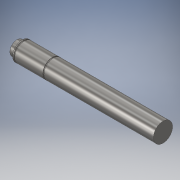
# Autodesk Inventor part: Main Axle
Saved by Autodesk Inventor 2019.4 (Build 234330000, 330)
## iProperties
Created: 2019-11-02
Part Number: Main Axle
Material: Stainless Steel
Document SubType Name: Modeling
Designer: admin
Density: 8 g/cm^3
Appearance: Semi-Polished
Author: admin
Autodesk Inventor part; units mm, degrees
ref_plane "YZ Plane" through (0, 0, 0) normal (1, 0, 0) x (0, 1, 0)
ref_plane "XZ Plane" through (0, 0, 0) normal (0, 1, 0) x (-1, 0, 0)
ref_plane "XY Plane" through (0, 0, 0) normal (0, 0, 1) x (1, 0, 0)
sketch "Sketch1" plane through (0, 0, 0) normal (0, 1, 0) x (-1, 0, 0)
  line L0 (0, 0) -> (0, -7.3)
  line L1 (0, -7.3) -> (-5.3, -7.3)
  line L2 (-5.3, -7.3) -> (-5.3, -9.8)
  line L3 (-150, -9.8) -> (-150, 0)
  line L4 (-150, 0) -> (0, 0)
  line L5 (-5.3, -9.8) -> (-6.4, -9.8)
  line L6 (-6.4, -9.8) -> (-6.4, -9.3)
  line L7 (-6.4, -9.3) -> (-7.5, -9.3)
  line L8 (-7.5, -9.3) -> (-7.5, -9.8)
  line L9 (-7.5, -9.8) -> (-36.4, -9.8)
  line L10 (-36.4, -9.8) -> (-36.4, -9.3)
  line L11 (-36.4, -9.3) -> (-37.5, -9.3)
  line L12 (-37.5, -9.3) -> (-37.5, -9.8)
  line L13 (-37.5, -9.8) -> (-150, -9.8)
  dimension "d0" = 5.3
  dimension "d1" = 7.3
  dimension "d3" = 1.1
  dimension "d4" = 0.5
  dimension "d5" = 9.8
  dimension "d6" = 6.4
  dimension "d7" = 1.1
  dimension "d8" = 36.4
  dimension "d9" = 150
  constraints: 28 end point, 9 perpendicular, 5 point on line, 1 horizontal, 1 vertical
  measures "d0" distance of L0.end L1.end
  measures "d1" distance of L0.start L0.end
  measures "d3" distance of L6.end L7.end
  measures "d4" distance of L5.end L6.end
  measures "d5" distance between parallel lines of L4 L5
  measures "d6" distance between parallel lines of L0 L6
  measures "d7" distance of L10.end L11.end
  measures "d8" distance between parallel lines of L0 L10
  measures "d9" distance of L3.end L0.start
revolve "Revolution1" add sketch "Sketch1" angle 360 about axis through (150, 0, 0) along (-1, 0, 0)
body "Solid1"
